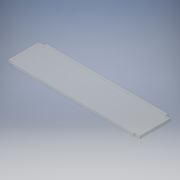
# Autodesk Inventor part: SeitenOben
Saved by Autodesk Inventor 2016 (Build 200138000, 138)
## iProperties
Created: 2018-04-27
Part Number: SeitenOben
Material: Polycarbonate, Clear
Document SubType Name: Modeling
Designer: Phil Erle
Density: 1.2 g/cm^3
Appearance: Polycarbonate - Clear
Author: Phil Erle
Autodesk Inventor part; units mm, degrees
ref_plane "YZ Plane" through (0, 0, 0) normal (1, 0, 0) x (0, 1, 0)
ref_plane "XZ Plane" through (0, 0, 0) normal (0, 1, 0) x (-1, 0, 0)
ref_plane "XY Plane" through (0, 0, 0) normal (0, 0, 1) x (1, 0, 0)
sketch "Sketch1" plane through (0, 0, 0) normal (0, 0, 1) x (1, 0, 0)
  line L0 (-130, 30) -> (-130, -30)
  line L1 (-130, -30) -> (-120, -30)
  line L2 (-120, -30) -> (-120, -32.5)
  line L3 (-120, -32.5) -> (120, -32.5)
  line L4 (120, -32.5) -> (120, -30)
  line L5 (120, -30) -> (130, -30)
  line L6 (130, -30) -> (130, 30)
  line L7 (130, 30) -> (120, 30)
  line L8 (120, 30) -> (120, 35)
  line L9 (120, 35) -> (-120, 35)
  line L10 (-120, 35) -> (-120, 30)
  line L11 (-130, 30) -> (-120, 30)
  point P0 (0, 0)
  point P1 (0, 35)
  point P2 (130, 0)
  point P3 (-130, 0)
  dimension "d0" = 5
  dimension "d1" = 240
  dimension "d2" = 10
  dimension "d3" = 10
  dimension "d4" = 2.5
  dimension "d5" = 60
  constraints: 24 end point, 8 perpendicular, 7 point on line, 3 midpoint, 1 horizontal alignment, 1 vertical, 1 vertical alignment
  measures "d0" distance of L7.end L8.end
  measures "d1" distance of L8.end L9.end
  measures "d2" distance of L0.start L10.end
  measures "d3" distance of L6.end L7.end
  measures "d4" distance of L3.end L4.end
  measures "d5" distance between parallel lines of L1 L11
extrude "Extrusion1" add sketch "Sketch1" along normal blind 5
body "Solid1"
